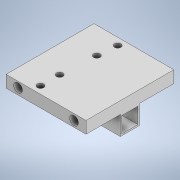
# Autodesk Inventor part: fuselage_wing_interface
Saved by Autodesk Inventor 2021 (Build 250183000, 183)
## iProperties
Created: 2020-11-15
Part Number: fuselage_wing_interface
Material: Generic
Document SubType Name: Modeling
Designer: Paco
Density: 1 g/cm^3
Appearance: Default
Author: Paco
Autodesk Inventor part; units mm, degrees
ref_plane "YZ Plane" through (0, 0, 0) normal (1, 0, 0) x (0, 1, 0)
ref_plane "XZ Plane" through (0, 0, 0) normal (0, 1, 0) x (-1, 0, 0)
sketch "Sketch1" plane through (0, 0, 0) normal (1, 0, 0) x (0, 1, 0)
  line L0 (2.9838, 8.2524) -> (-9.0162, 8.2524)
  line L1 (-9.0162, 8.2524) -> (-9.0162, -3.7476)
  line L2 (-9.0162, -3.7476) -> (2.9838, -3.7476)
  line L3 (2.9838, -3.7476) -> (2.9838, 8.2524)
  line L4 (1.9838, 7.2524) -> (-8.0162, 7.2524)
  line L5 (-8.0162, 7.2524) -> (-8.0162, -2.7476)
  line L6 (-8.0162, -2.7476) -> (1.9838, -2.7476)
  line L7 (1.9838, -2.7476) -> (1.9838, 7.2524)
  line L8 (10.4838, 29.7524) -> (2.9838, 29.7524)
  line L9 (2.9838, 29.7524) -> (2.9838, -25.2476)
  line L10 (2.9838, -25.2476) -> (10.4838, -25.2476)
  line L11 (10.4838, -25.2476) -> (10.4838, 29.7524)
  point P0 (0, 0)
  dimension "d0" = 12
  dimension "d1" = 10
  dimension "d2" = 10
  dimension "d3" = 12
  dimension "d4" = 1
  dimension "d5" = 1
  dimension "d22" = 21.5
  dimension "d24" = 55
  dimension "d25" = 7.5
  dimension "d55" = 21.5
  constraints: 24 end point, 6 parallel, 3 horizontal, 3 perpendicular, 1 collinear
  measures "d0" distance of L2.end L0.start
  measures "d1" distance of L6.end L4.start
  measures "d2" distance of L4.start L4.end
  measures "d3" distance of L1.end L2.end
  measures "d4" distance between parallel lines of L3 L7
  measures "d5" distance between parallel lines of L2 L6
  measures "d22" distance between parallel lines of L0 L8
  measures "d24" distance of L10.end L8.start
  measures "d25" distance of L9.end L10.end
  measures "d55" distance between parallel lines of L10 L2
extrude "Extrusion1" add sketch "Sketch1" along normal blind 50
ref_plane "Work Plane1" through (0, -9.0162, 2.2524) normal (0, 0, 1) x (1, 0, 0)
sketch "Sketch3" plane through (0, 2.9838, 29.7524) normal (0, 0, 1) x (1, 0, 0)
  line L0 (50, 7.5) -> (50, 0) projected
  line L1 (0, 7.5) -> (50, 7.5) projected
  point P0 (0, -2.9838)
  point P1 (7.5006, 3.9603)
  point P2 (42.5, 3.75)
  dimension "d26" = 35
  dimension "d27" = 7.5
  dimension "d28" = 50
  dimension "d29" = 7.5
  dimension "d30" = 3.75
  measures "d26" distance of point (42.5, 3.75) point (7.501, 3.96)
  measures "d27" distance from line of L0 point (42.5, 3.75)
  measures "d28" distance of L1.start L0.start
  measures "d29" distance of L0.start L0.end
  measures "d30" distance from line of L1 point (42.5, 3.75)
hole "Hole1" at (42.5, 6.7338, 29.7524) at (7.5006, 6.944, 29.7524) direction (0, 0, -1) diameter 5.5 end through all
sketch "Sketch4" plane through (0, 10.4838, 29.7524) normal (0, 1, 0) x (1, 0, 0)
  line L0 (50, 55) -> (50, 0) projected
  line L1 (0, 0) -> (50, 0) projected
  line L2 (50, 21.5) -> (50, 33.5) projected
  line L3 (0, 55) -> (0, 0) projected
  line L4 (0, 55) -> (50, 55) projected
  point P0 (0, 29.7524)
  point P1 (17, 4.5)
  point P2 (17, 16.5)
  point P3 (19.3365, 50.5)
  point P4 (18.2576, 38.5)
  dimension "d38" = 33
  dimension "d39" = 4.5
  dimension "d40" = 12
  dimension "d57" = 12
  dimension "d58" = 4.5
  measures "d38" distance from line of L0 point (17, 4.5)
  measures "d39" distance from line of L1 point (17, 4.5)
  measures "d40" distance of point (17, 4.5) point (17, 16.5)
  measures "d57" vertical distance of point (19.337, 50.5) point (18.258, 38.5)
  measures "d58" distance from line of point (19.337, 50.5) L4
hole "Hole3" at (19.3365, 10.4838, -20.7476) at (18.2576, 10.4838, -8.7476) at (17, 10.4838, 13.2524) at (17, 10.4838, 25.2524) direction (0, -1, 0) diameter 4 end through all
equation "\"d2\" = d1"
equation "\"d3\" = d0"
equation "\"d5\" = d4"
equation "\"d22\" = d55"
equation "\"d27\" = -0.5 * d26 + 0.5 * d28"
equation "\"d30\" = 0.5 * d29"
equation "\"d57\" = d40"
equation "\"d58\" = d39"
body "Solid1"
